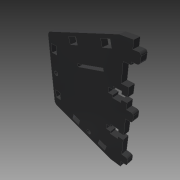
# Autodesk Inventor part: front_panel_2004_brace_left
Saved by Autodesk Inventor 2014 (Build 180170000, 170)
## iProperties
Created: 2014-01-11
Part Number: front_panel_2004_brace_left
Material: Generic
Document SubType Name: Modeling
Designer: buben
Density: 1 g/cm^3
Appearance: Anodized - Dark Gray
Author: buben
Autodesk Inventor part; units mm, degrees
ref_plane "YZ Plane" through (0, 0, 0) normal (1, 0, 0) x (0, 1, 0)
ref_plane "XZ Plane" through (0, 0, 0) normal (0, 1, 0) x (-1, 0, 0)
ref_plane "XY Plane" through (0, 0, 0) normal (0, 0, 1) x (1, 0, 0)
sketch "Sketch1" plane through (0, 0, 0) normal (0, 1, 0) x (-1, 0, 0)
  line L0 (0, 108) -> (0, 0)
  line L1 (0, 0) -> (10.412, 0)
  line L2 (10.412, 0) -> (80.1677, 18.691)
  line L3 (80.1677, 18.691) -> (80.1677, 89.309)
  line L4 (80.1677, 89.309) -> (10.412, 108)
  line L5 (10.412, 108) -> (0, 108)
  line L6 (2.5529, 107) -> (1, 101.2044) construction
  line L7 (1, 101.2044) -> (68.6148, 83.0871) construction
  line L8 (68.6148, 83.0871) -> (70.1677, 88.8827) construction
  line L9 (70.1677, 88.8827) -> (2.5529, 107) construction
  line L10 (1, 6.7956) -> (2.5529, 1) construction
  line L11 (2.5529, 1) -> (70.1677, 19.1173) construction
  line L12 (70.1677, 19.1173) -> (68.6148, 24.9129) construction
  line L13 (68.6148, 24.9129) -> (1, 6.7956) construction
  line L14 (71.1677, 88.309) -> (77.1677, 88.309) construction
  line L15 (77.1677, 88.309) -> (77.1677, 19.691) construction
  line L16 (77.1677, 19.691) -> (71.1677, 19.691) construction
  line L17 (71.1677, 19.691) -> (71.1677, 88.309) construction
  line L18 (17.0418, 103.1177) -> (15.4889, 97.3222)
  line L19 (15.4889, 97.3222) -> (23.2163, 95.2516)
  line L20 (23.2163, 95.2516) -> (24.7692, 101.0472)
  line L21 (24.7692, 101.0472) -> (17.0418, 103.1177)
  line L22 (47.9514, 94.8355) -> (46.3985, 89.0399)
  line L23 (46.3985, 89.0399) -> (54.1259, 86.9694)
  line L24 (54.1259, 86.9694) -> (55.6788, 92.765)
  line L25 (55.6788, 92.765) -> (47.9514, 94.8355)
  line L26 (15.4889, 10.6778) -> (17.0418, 4.8823)
  line L27 (17.0418, 4.8823) -> (24.7692, 6.9528)
  line L28 (24.7692, 6.9528) -> (23.2163, 12.7484)
  line L29 (23.2163, 12.7484) -> (15.4889, 10.6778)
  line L30 (46.3985, 18.9601) -> (47.9514, 13.1645)
  line L31 (47.9514, 13.1645) -> (55.6788, 15.235)
  line L32 (55.6788, 15.235) -> (54.1259, 21.0306)
  line L33 (54.1259, 21.0306) -> (46.3985, 18.9601)
  line L34 (54.9024, 89.8672) -> (69.3913, 85.9849) construction
  line L35 (16.2653, 7.7801) -> (1.7765, 3.8978) construction
  line L36 (54.9024, 18.1328) -> (69.3913, 22.0151) construction
  line L37 (16.2653, 100.2199) -> (1.7765, 104.1022) construction
  line L38 (71.1677, 80.309) -> (77.1677, 80.309)
  line L39 (77.1677, 80.309) -> (77.1677, 72.309)
  line L40 (77.1677, 72.309) -> (71.1677, 72.309)
  line L41 (71.1677, 72.309) -> (71.1677, 80.309)
  line L42 (71.1677, 35.691) -> (77.1677, 35.691)
  line L43 (77.1677, 35.691) -> (77.1677, 27.691)
  line L44 (77.1677, 27.691) -> (71.1677, 27.691)
  line L45 (71.1677, 27.691) -> (71.1677, 35.691)
  line L46 (74.1677, 80.309) -> (74.1677, 88.309) construction
  line L47 (74.1677, 27.691) -> (74.1677, 19.691) construction
  dimension "d0" = 70
  dimension "d1" = 6
  dimension "d3" = 70
  dimension "d4" = 6
  dimension "d7" = 3
  dimension "d8" = 3
  dimension "d9" = 6
  dimension "d10" = 3
  dimension "d11" = 1
  dimension "d12" = 1
  dimension "d13" = 1
  dimension "d14" = 1
  dimension "d15" = 15
  dimension "d16" = 1
  dimension "d17" = 1
  dimension "d18" = 1
  dimension "d19" = 108
  dimension "d20" = 8
  dimension "d21" = 15
  dimension "d22" = 8
  constraints: 96 end point, 21 parallel, 15 perpendicular, 12 midpoint, 12 point on line, 9 equal length, 3 horizontal, 1 vertical, 1 vertical alignment
  measures "d0" distance of L6.end L7.end
  measures "d1" distance of L7.end L8.end
  measures "d3" distance of L12.end L10.start
  measures "d4" distance of L11.end L12.end
  measures "d7" distance between parallel lines of L4 L9
  measures "d8" distance between parallel lines of L2 L11
  measures "d9" distance of L14.start L14.end
  measures "d10" distance between parallel lines of L3 L15
  measures "d11" distance from line of L0 L6.end
  measures "d12" distance from line of L0 L10.start
  measures "d13" distance from line of L6.start L5
  measures "d14" distance from line of L1 L10.end
  measures "d15" angle of L5 L4
  measures "d16" distance from line of L3.end L14
  measures "d17" horizontal distance of L14.start L8.end
  measures "d18" distance from line of L2.end L16
  measures "d19" distance of L0.start L0.end
  measures "d20" distance between parallel lines of L20 L18
  measures "d21" distance of L37.start L37.end
  measures "d22" distance of L47.start L47.end
extrude "Extrusion7" add sketch "Sketch1" along normal blind 6
sketch "Sketch7" plane through (0, 0, 0) normal (0, -1, 0) x (1, 0, 0)
  line L0 (0, 0) -> (0, 108) projected
  line L1 (0, 92) -> (-6, 92)
  line L2 (-6, 92) -> (-6, 76)
  line L3 (-6, 76) -> (0, 76)
  line L4 (0, 76) -> (0, 92)
  dimension "d74" = 16
  dimension "d75" = 16
  dimension "d76" = 6
  constraints: 8 end point, 2 parallel, 1 horizontal, 1 perpendicular, 1 point on line
  measures "d74" distance of L1.end L2.end
  measures "d75" distance from line of L1 L0.end
  measures "d76" distance of L2.end L3.end
extrude "Extrusion8" cut sketch "Sketch7" against normal blind 6
sketch "Sketch8" plane through (0, 0, 0) normal (0, -1, 0) x (1, 0, 0)
  line L0 (-77.1677, 72.309) -> (-71.1677, 35.691) construction
  line L1 (-77.1677, 35.691) -> (-71.1677, 72.309) construction
  circle A0 centre (-74.1677, 54) radius 2.25
  dimension "d80" = 4.5
  constraints: 4 end point, 1 centre point, 1 midpoint
  measures "d80" diameter of A0
extrude "Extrusion9" cut sketch "Sketch8" against normal blind 6
sketch "Sketch9" plane through (0, 0, 0) normal (0, -1, 0) x (1, 0, 0)
  line L0 (-46.3985, 18.9601) -> (-24.7692, 6.9528) construction
  line L1 (-23.2163, 12.7484) -> (-47.9514, 13.1645) construction
  circle A0 centre (-35.5839, 12.9564) radius 2.25
  dimension "d83" = 4.5
  constraints: 4 end point, 1 centre point, 1 midpoint
  measures "d83" diameter of A0
extrude "Extrusion10" cut sketch "Sketch9" against normal blind 6
sketch "Sketch10" plane through (0, 0, 0) normal (0, -1, 0) x (1, 0, 0)
  line L0 (0, 0) -> (0, 76) projected
  line L1 (0, 68.25) -> (0, 63.75)
  line L2 (-16.3, 63.75) -> (-16.3, 68.25)
  line L3 (-12.3, 70.75) -> (-5, 70.75)
  line L4 (-5, 61.25) -> (-12.3, 61.25)
  line L5 (-16.3, 68.25) -> (-12.3, 68.25)
  line L6 (-5, 68.25) -> (0, 68.25)
  line L7 (0, 63.75) -> (-5, 63.75)
  line L8 (-12.3, 63.75) -> (-16.3, 63.75)
  line L9 (-12.3, 61.25) -> (-12.3, 63.75)
  line L10 (-12.3, 68.25) -> (-12.3, 70.75)
  line L11 (-5, 70.75) -> (-5, 68.25)
  line L12 (-5, 63.75) -> (-5, 61.25)
  line L13 (0, 34.25) -> (0, 29.75)
  line L14 (-16.3, 29.75) -> (-16.3, 34.25)
  line L15 (-12.3, 36.75) -> (-5, 36.75)
  line L16 (-5, 27.25) -> (-12.3, 27.25)
  line L17 (-16.3, 34.25) -> (-12.3, 34.25)
  line L18 (-5, 34.25) -> (0, 34.25)
  line L19 (0, 29.75) -> (-5, 29.75)
  line L20 (-12.3, 29.75) -> (-16.3, 29.75)
  line L21 (-12.3, 27.25) -> (-12.3, 29.75)
  line L22 (-12.3, 34.25) -> (-12.3, 36.75)
  line L23 (-5, 36.75) -> (-5, 34.25)
  line L24 (-5, 29.75) -> (-5, 27.25)
  point P0 (0, 108)
  point P1 (-16.3, 66)
  point P2 (-16.3, 32)
  dimension "d86" = 4.5
  dimension "d87" = 2.5
  dimension "d88" = 2.5
  dimension "d89" = 5
  dimension "d90" = 7.3
  dimension "d91" = 4
  dimension "d92" = 4.5
  dimension "d93" = 2.5
  dimension "d94" = 2.5
  dimension "d95" = 5
  dimension "d96" = 7.3
  dimension "d97" = 4
  dimension "d98" = 42
  dimension "d99" = 34
  constraints: 48 end point, 20 parallel, 10 collinear, 8 perpendicular, 6 horizontal, 2 midpoint
  measures "d86" distance of L2.start L2.end
  measures "d87" distance of L5.end L3.start
  measures "d88" distance of L4.end L8.start
  measures "d89" distance of L6.start L1.start
  measures "d90" distance of L3.start L3.end
  measures "d91" distance of L2.end L5.end
  measures "d92" distance of L14.start L14.end
  measures "d93" distance of L22.start L22.end
  measures "d94" distance of L21.start L21.end
  measures "d95" distance of L23.end L13.start
  measures "d96" distance of L22.end L15.end
  measures "d97" distance of L14.end L22.start
  measures "d98" vertical distance of point (-16.3, 66) point (0, 108)
  measures "d99" distance of point (-16.3, 32) point (-16.3, 66)
extrude "Extrusion11" cut sketch "Sketch10" against normal blind 6
sketch "Sketch11" plane through (0, 0, 0) normal (0, -1, 0) x (1, 0, 0)
  line L0 (0, 68.25) -> (0, 76) projected
  line L1 (0, 108) -> (-10.412, 108) projected
  line L2 (-23.2163, 95.2516) -> (-24.7692, 101.0472) projected
  line L3 (-46.4441, 73.7575) -> (-22.296, 80.228) construction
  line L4 (-22.296, 80.228) -> (-21.9078, 78.7791) construction
  line L5 (-21.9078, 78.7791) -> (-46.0559, 72.3086) construction
  line L6 (-46.0559, 72.3086) -> (-46.4441, 73.7575) construction
  line L7 (-47.0565, 74.1111) -> (-21.9424, 80.8404)
  line L8 (-21.9424, 80.8404) -> (-21.2954, 78.4256)
  line L9 (-21.2954, 78.4256) -> (-46.4095, 71.6963)
  line L10 (-46.4095, 71.6963) -> (-47.0565, 74.1111)
  dimension "d102" = 25
  dimension "d103" = 1.5
  dimension "d104" = 0.5
  dimension "d105" = 22.296
  dimension "d106" = 27.772
  constraints: 16 end point, 4 parallel, 3 perpendicular, 3 other
  measures "d102" distance of L4.end L5.end
  measures "d103" distance of L5.end L3.start
  measures "d104" distance between parallel lines of L9 L5
  measures "d105" distance from line of L0 L3.end
  measures "d106" distance from line of L1 L3.end
extrude "Extrusion12" cut sketch "Sketch11" against normal blind 6
chamfer "Chamfer2" distance 2 angle 45 2 edges at (-80.1677, 3, 89.309) (-80.1677, 3, 18.691)
sketch "Sketch12" plane through (0, 0, 0) normal (0, -1, 0) x (1, 0, 0)
  line L0 (0, 0) -> (0, 29.75) projected
  line L1 (0, 34.25) -> (0, 63.75) projected
  line L2 (0, 92) -> (0, 108) projected
  line L3 (0, 108) -> (-10.412, 108) projected
  line L4 (0, 102) -> (4, 102)
  line L5 (6, 100) -> (6, 96)
  line L6 (4, 94) -> (0, 94)
  line L7 (0, 94) -> (0, 102)
  line L8 (0, 58) -> (4, 58)
  line L9 (6, 56) -> (6, 52)
  line L10 (4, 50) -> (0, 50)
  line L11 (0, 50) -> (0, 58)
  line L12 (0, 14) -> (4, 14)
  line L13 (6, 12) -> (6, 8)
  line L14 (4, 6) -> (0, 6)
  line L15 (0, 6) -> (0, 14)
  arc A0 (6, 100) -> (4, 102) centre (4, 100) ccw
  arc A1 (4, 94) -> (6, 96) centre (4, 96) ccw
  arc A2 (6, 56) -> (4, 58) centre (4, 56) ccw
  arc A3 (4, 50) -> (6, 52) centre (4, 52) ccw
  arc A4 (4, 6) -> (6, 8) centre (4, 8) ccw
  arc A5 (6, 12) -> (4, 14) centre (4, 12) ccw
  dimension "d112" = 2
  dimension "d113" = 8
  dimension "d114" = 8
  dimension "d115" = 8
  dimension "d116" = 6
  dimension "d117" = 6
  dimension "d118" = 36
  dimension "d119" = 36
  constraints: 24 end point, 12 point on circle, 12 tangent, 6 centre point, 6 parallel, 5 equal radius, 3 horizontal, 3 perpendicular, 3 point on line, 2 collinear
  measures "d112" radius of A0
  measures "d113" distance between parallel lines of L6 L4
  measures "d114" distance between parallel lines of L10 L8
  measures "d115" distance between parallel lines of L12 L14
  measures "d116" distance between parallel lines of L2 L5
  measures "d117" distance between parallel lines of L3 L4
  measures "d118" distance between parallel lines of L8 L6
  measures "d119" distance between parallel lines of L12 L10
extrude "Extrusion13" add sketch "Sketch12" against normal blind 6
equation "\"d3\" = d0"
equation "\"d4\" = d1"
equation "\"d8\" = d7"
equation "\"d9\" = d1"
equation "\"d10\" = d7"
equation "\"d12\" = d11"
equation "\"d88\" = d87"
equation "\"d94\" = d93"
body "Solid2"
